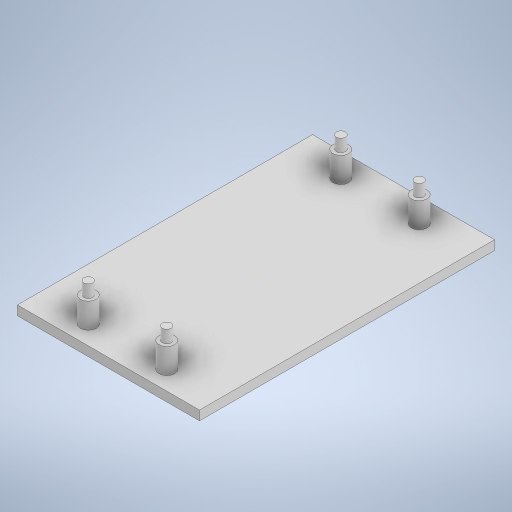
# Autodesk Inventor part: drzak_plos
Saved by Autodesk Inventor 2024 (Build 280153000, 153)
## iProperties
Created: 2025-02-19
Part Number: drzak_plos
Material: Všeobecné
Document SubType Name: Modeling
Designer: eliasla
Density: 1 g/cm^3
Appearance: Výchozí
Author: eliasla
Autodesk Inventor part; units mm, degrees
ref_plane "YZ Plane" through (0, 0, 0) normal (1, 0, 0) x (0, 1, 0)
ref_plane "XZ Plane" through (0, 0, 0) normal (0, 1, 0) x (-1, 0, 0)
ref_plane "XY Plane" through (0, 0, 0) normal (0, 0, 1) x (1, 0, 0)
sketch "Náčrt1" plane through (0, 0, 0) normal (0, 0, 1) x (1, 0, 0)
  line L0 (-29, -47) -> (29, -47)
  line L1 (29, -47) -> (29, 47)
  line L2 (29, 47) -> (-29, 47)
  line L3 (-29, 47) -> (-29, -47)
  line L4 (-29, -47) -> (29, 47) construction
  line L5 (29, -47) -> (-29, 47) construction
  line L6 (0, 47) -> (0, -47)
  line L7 (0, -43.9165) -> (12.5, -43.9165)
  point P0 (0, 0)
  dimension "d0" = 58
  dimension "d1" = 94
  dimension "d2" = 12.5
  constraints: 16 end point, 4 midpoint, 2 horizontal, 2 parallel, 1 perpendicular, 1 point on line
  measures "d0" distance of L1.end L2.end
  measures "d1" distance of L0.end L1.end
  measures "d2" distance of L7.start L7.end
extrude "Vysunutí1" add sketch "Náčrt1" along normal blind 3
sketch "Náčrt2" plane through (0, 0, 3) normal (0, 0, 1) x (1, 0, 0)
  point P0 (0, 0)
sketch "Náčrt3" plane through (0, 0, 3) normal (0, 0, 1) x (1, 0, 0)
  line L0 (0, -40.9336) -> (12.5, -40.9336)
  circle A0 centre (12.5, -40.9336) radius 1.45
  line L1 (0, 0) -> (0, -12.3388)
  circle A1 centre (-12.5, -40.9336) radius 1.45
  line L2 (-12.5, -39.4836) -> (-12.5, 38.0164)
  circle A2 centre (-12.5, 39.5164) radius 1.45
  circle A3 centre (12.5, 39.5164) radius 1.45
  dimension "d5" = 12.5
  dimension "d6" = 2.9
  dimension "d7" = 77.5
  dimension "d8" = 2.9
  dimension "d9" = 1.5
  constraints: 6 end point, 3 centre point, 2 symmetric about line, 2 vertical, 1 coincident, 1 horizontal, 1 vertical alignment, 4 other
  measures "d5" distance of L0.start L0.end
  measures "d6" diameter of A0
  measures "d7" distance of L2.start L2.end
  measures "d8" diameter of A2
  measures "d9" distance of L2.end A2.centre
extrude "Vysunutí2" add sketch "Náčrt3" along normal blind 12
sketch "Náčrt4" plane through (0, 0, 3) normal (0, 0, 1) x (1, 0, 0)
  circle A0 centre (12.5, 39.5164) radius 1.45 projected
  circle A1 centre (12.5, 39.5164) radius 2.5
  circle A2 centre (-12.5, 39.5164) radius 1.45 projected
  circle A3 centre (-12.5, 39.5164) radius 2.5
  circle A4 centre (-12.5, -40.9336) radius 1.45 projected
  circle A5 centre (-12.5, -40.9336) radius 2.5
  circle A6 centre (12.5, -40.9336) radius 1.45 projected
  circle A7 centre (12.5, -40.9336) radius 2.5
  point P0 (0, 0)
  dimension "d12" = 5
  dimension "d13" = 5
  dimension "d14" = 5
  dimension "d15" = 5
  constraints: 4 centre point, 4 coincident
  measures "d12" diameter of A1
  measures "d13" diameter of A3
  measures "d14" diameter of A5
  measures "d15" diameter of A7
extrude "Vysunutí3" add sketch "Náčrt4" along normal blind 8 contours A0 | A1 | A2 | A3 | A4 | A5 | A6 | A7
